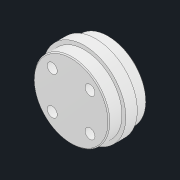
# Autodesk Inventor part: scara-base6
Saved by Autodesk Inventor 2022 (Build 260153000, 153)
## iProperties
Created: 2021-10-10
Part Number: scara-base6
Material: ABS プラスチック
Document SubType Name: Modeling
Designer: Yuta Kage
Density: 1.06 g/cm^3
Appearance: 滑らか - 白
Description: 印刷
Mass: 17.3059 g
Surface Area: 49.5423 cm^2
Volume: 16.3263 cm^3
Author: Yuta Kage
Autodesk Inventor part; units mm, degrees
ref_plane "YZ Plane" through (0, 0, 0) normal (1, 0, 0) x (0, 1, 0)
ref_plane "XZ Plane" through (0, 0, 0) normal (0, 1, 0) x (-1, 0, 0)
ref_plane "XY Plane" through (0, 0, 0) normal (0, 0, 1) x (1, 0, 0)
sketch "スケッチ1" plane through (0, 0, 0) normal (1, 0, 0) x (0, 1, 0)
  line L0 (0, 0) -> (20, 0)
  line L1 (20, -20) -> (0, -20)
  line L2 (0, -20) -> (0, 0)
  line L3 (20, 0) -> (20, -6.95)
  line L4 (20, -6.95) -> (22, -6.95)
  line L5 (22, -6.95) -> (22, -13.05)
  line L6 (22, -13.05) -> (20, -13.05)
  line L7 (20, -13.05) -> (20, -20)
  point P0 (12, 0)
  dimension "d0" = 20
  dimension "d34" = 2
  dimension "d35" = 6.95
  dimension "d36" = 20
  dimension "d37" = 6.95
  constraints: 16 end point, 5 perpendicular, 2 point on line, 1 horizontal, 1 vertical
  measures "d0" distance of L0.start L0.end
  measures "d34" distance of L5.end L6.end
  measures "d35" distance of L0.end L3.end
  measures "d36" distance between parallel lines of L1 L0
  measures "d37" distance of L6.end L1.start
revolve "回転1" add sketch "スケッチ1" angle 360 about axis through (0, 0, -20) along (0, 0, 1)
chamfer "面取り1" distance 0.5 angle 45 2 edges at (0, -20, 0) (0, -20, -20)
sketch "スケッチ4" plane through (0, 0, -20) normal (0, 0, -1) x (-1, 0, 0)
  line L0 (-10, 10) -> (10, 10)
  line L1 (10, 10) -> (10, -10)
  line L2 (10, -10) -> (-10, -10)
  line L3 (-10, -10) -> (-10, 10)
  line L4 (-10, 10) -> (10, -10) construction
  line L5 (10, 10) -> (-10, -10) construction
  point P0 (0, 0)
  dimension "d24" = 20
  dimension "d25" = 20
  constraints: 12 end point, 2 midpoint, 2 parallel, 1 horizontal, 1 perpendicular
  measures "d24" distance of L1.end L2.end
  measures "d25" distance of L0.end L1.end
hole "穴2" at (-10, 10, -20) at (-10, -10, -20) at (10, -10, -20) at (10, 10, -20) direction (0, 0, 1) diameter 5.3 end through all clearance for "Socket Head Cap Screw" size "M5" standard "Ansi Metric M Profile"
ref_plane "作業平面1" through (0, 0, -10) normal (0, 0, 1) x (1, 0, 0)
equation "\"d37\" = d35"
